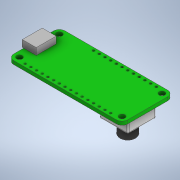
# Autodesk Inventor part: ESP8266 Feather
Saved by Autodesk Inventor 2021 (Build 250183000, 183)
## iProperties
Created: 2022-02-21
Part Number: ESP8266 Feather
Material: Generic
Document SubType Name: Modeling
Designer: maxsm
Density: 1 g/cm^3
Appearance: Default
Author: maxsm
Autodesk Inventor part; units mm, degrees
ref_plane "YZ Plane" through (0, 0, 0) normal (1, 0, 0) x (0, 1, 0)
ref_plane "XZ Plane" through (0, 0, 0) normal (0, 1, 0) x (-1, 0, 0)
ref_plane "XY Plane" through (0, 0, 0) normal (0, 0, 1) x (1, 0, 0)
sketch "Sketch1" plane through (0, 0, 0) normal (0, 1, 0) x (-1, 0, 0)
  line L0 (22.86, 11.43) -> (-22.86, 11.43)
  line L1 (-25.4, 8.89) -> (-25.4, -8.89)
  line L2 (-22.86, -11.43) -> (22.86, -11.43)
  line L3 (25.4, -8.89) -> (25.4, 8.89)
  line L4 (25.4, 11.43) -> (-25.4, -11.43) construction
  line L5 (-25.4, 11.43) -> (25.4, -11.43) construction
  circle A0 centre (22.86, 8.89) radius 1.27
  circle A1 centre (22.86, -8.89) radius 1.27
  circle A2 centre (-22.86, 8.89) radius 1.27
  circle A3 centre (-22.86, -8.89) radius 1.27
  arc A4 (25.4, 8.89) -> (22.86, 11.43) centre (22.86, 8.89) ccw
  arc A5 (22.86, -11.43) -> (25.4, -8.89) centre (22.86, -8.89) ccw
  arc A6 (-22.86, 11.43) -> (-25.4, 8.89) centre (-22.86, 8.89) ccw
  arc A7 (-25.4, -8.89) -> (-22.86, -11.43) centre (-22.86, -8.89) ccw
  point P0 (0, 0)
  dimension "d0" = 50.8
  dimension "d1" = 22.86
  dimension "d2" = 2.54
  dimension "d6" = 17.78
  dimension "d9" = 8.89
  dimension "d10" = 2.54
  dimension "d11" = 2.54
  dimension "d13" = 2.54
  dimension "d14" = 2.54
  dimension "d15" = 2.54
  constraints: 12 end point, 8 centre point, 8 point on circle, 8 point on line, 8 tangent, 6 equal radius, 2 horizontal alignment, 2 midpoint, 2 parallel, 1 horizontal, 1 perpendicular
  measures "d0" distance of L5.end L4.end
  measures "d1" distance of L4.end L5.start
  measures "d2" diameter of A0
  measures "d6" distance of A1.centre A0.centre
  measures "d9" vertical distance of A0.centre point (0, 0)
  measures "d10" distance from line of A0.centre L3
  measures "d11" distance from line of L3 A1.centre
  measures "d13" distance from line of L1 A3.centre
  measures "d14" distance from line of L1 A2.centre
  measures "d15" radius of A4
extrude "Extrusion1" add sketch "Sketch1" along normal blind 1.6
sketch "Sketch4" plane through (0, 1.6, 0) normal (0, 1, 0) x (1, 0, 0)
  line L0 (-19.812, -4.445) -> (-26.035, -4.445)
  line L1 (-26.035, -4.445) -> (-26.035, 4.445)
  line L2 (-26.035, 4.445) -> (-19.812, 4.445)
  line L3 (-19.812, 4.445) -> (-19.812, -4.445)
  line L4 (-19.812, -4.445) -> (-26.035, 4.445) construction
  line L5 (-26.035, -4.445) -> (-19.812, 4.445) construction
  line L6 (-25.4, 8.89) -> (-25.4, -8.89) projected
  line L7 (-36.322, 0) -> (35.687, 0) projected
  point P0 (0, 0)
  point P1 (-22.9235, 0)
  dimension "d34" = 0.635
  dimension "d35" = 6.223
  dimension "d62" = 8.89
  constraints: 12 end point, 2 midpoint, 2 parallel, 1 horizontal, 1 perpendicular, 1 other
  measures "d34" distance between parallel lines of L6 L1
  measures "d35" distance between parallel lines of L1 L3
  measures "d62" distance between parallel lines of L0 L2
extrude "Extrusion4" add sketch "Sketch4" along normal blind 3
sketch "Sketch6" plane through (0, 1.6, 0) normal (0, 1, 0) x (1, 0, 0)
  circle A0 centre (-1.27, -10.16) radius 0.5
  line L0 (-22.86, -11.43) -> (22.86, -11.43) projected
  point P0 (0, 0)
  dimension "d46" = 1
  dimension "d47" = 1.27
  dimension "d48" = 1.27
  constraints: 1 centre point
  measures "d46" diameter of A0
  measures "d47" horizontal distance of A0.centre point (0, 0)
  measures "d48" distance from line of L0 A0.centre
extrude "Extrusion6" cut sketch "Sketch6" against normal through all
pattern_linear "Rectangular Pattern1" count 16 spacing 2.54 along (1, 0, 0) of "Extrusion6" first direction both ways yes
sketch "Sketch7" plane through (0, 1.6, 0) normal (0, 1, 0) x (1, 0, 0)
  circle A0 centre (3.81, 10.16) radius 0.5
  line L0 (-25.4, 8.89) -> (-25.4, 4.445) projected
  line L1 (22.86, 11.43) -> (-22.86, 11.43) projected
  point P0 (0, 0)
  point P1 (-10.668, 11.43)
  dimension "d54" = 29.21
  dimension "d55" = 1.27
  dimension "d56" = 1
  constraints: 1 centre point
  measures "d54" distance from line of L0 A0.centre
  measures "d55" distance from line of L1 A0.centre
  measures "d56" diameter of A0
extrude "Extrusion7" cut sketch "Sketch7" against normal through all
pattern_linear "Rectangular Pattern2" count 12 spacing 2.54 along (1, 0, 0) of "Extrusion7" first direction both ways yes
sketch "Sketch8" plane through (0, 0, 0) normal (0, -1, 0) x (1, 0, 0)
  line L0 (10.16, 6.35) -> (22.86, 6.35)
  line L1 (22.86, 6.35) -> (22.86, -6.35)
  line L2 (22.86, -6.35) -> (10.16, -6.35)
  line L3 (10.16, -6.35) -> (10.16, 6.35)
  line L4 (10.16, 6.35) -> (22.86, -6.35) construction
  line L5 (22.86, 6.35) -> (10.16, -6.35) construction
  line L6 (-25.4, -8.89) -> (-25.4, 8.89) projected
  point P0 (0, 0)
  point P1 (16.51, 0)
  point P2 (16.51, 0)
  dimension "d63" = 12.7
  dimension "d64" = 41.91
  constraints: 12 end point, 3 midpoint, 2 parallel, 2 perpendicular, 1 horizontal, 1 horizontal alignment
  measures "d63" distance between parallel lines of L2 L0
  measures "d64" distance from line of point (16.51, 0) L6
extrude "Extrusion8" add sketch "Sketch8" along normal blind 6.7
sketch "Sketch9" plane through (0, -6.7, 0) normal (0, -1, 0) x (1, 0, 0)
  circle A0 centre (16.51, 0) radius 3.556
  line L0 (10.16, -6.35) -> (10.16, 6.35) projected
  line L1 (10.16, 6.35) -> (22.86, 6.35) projected
  line L2 (22.86, 6.35) -> (22.86, -6.35) projected
  line L3 (22.86, -6.35) -> (10.16, -6.35) projected
  circle A1 centre (16.51, 0) radius 6.35
  point P0 (0, 0)
  dimension "d67" = 7.112
  constraints: 3 tangent, 2 centre point, 1 coincident
  measures "d67" diameter of A0
extrude "Extrusion9" add sketch "Sketch9" along normal blind 6.35 contours A0
fillet "Fillet2" radius 0.635 9 edges at (22.86, -3.35, 6.35) (10.16, -3.35, 6.35) (16.51, -6.7, 6.35) (22.86, -6.7, 0) (22.86, -3.35, -6.35) (16.51, -6.7, -6.35) (10.16, -6.7, 0) (10.16, -3.35, -6.35) (12.954, -13.05, 0)
sketch "Sketch10" plane through (0, 0, 0) normal (0, -1, 0) x (1, 0, 0)
  line L0 (-16.129, -4.064) -> (-8.001, -4.064)
  line L1 (-8.001, -4.064) -> (-8.001, 4.064)
  line L2 (-8.001, 4.064) -> (-16.129, 4.064)
  line L3 (-16.129, 4.064) -> (-16.129, -4.064)
  line L4 (-16.129, -4.064) -> (-8.001, 4.064) construction
  line L5 (-8.001, -4.064) -> (-16.129, 4.064) construction
  line L6 (-25.4, -8.89) -> (-25.4, 8.89) projected
  point P0 (0, 0)
  point P1 (-12.065, 0)
  point P2 (-12.065, 0)
  dimension "d72" = 8.128
  dimension "d74" = 13.335
  constraints: 12 end point, 3 midpoint, 2 parallel, 2 perpendicular, 1 horizontal, 1 horizontal alignment
  measures "d72" distance of L2.end L1.end
  measures "d74" distance from line of point (-12.065, 0) L6
extrude "Extrusion10" add sketch "Sketch10" along normal blind 3
sketch "Sketch11" plane through (0, -3, 0) normal (0, -1, 0) x (1, 0, 0)
  circle A0 centre (-12.065, 0) radius 1.27
  circle A1 centre (-12.065, 0) radius 4.064
  line L0 (-16.129, -4.064) -> (-8.001, -4.064) projected
  line L1 (-8.001, -4.064) -> (-8.001, 4.064) projected
  line L2 (-8.001, 4.064) -> (-16.129, 4.064) projected
  point P0 (0, 0)
  dimension "d77" = 2.54
  constraints: 3 tangent, 2 centre point, 1 concentric
  measures "d77" diameter of A0
extrude "Extrusion11" cut sketch "Sketch11" against normal blind 0.635 contours A0
body "Solid1"
